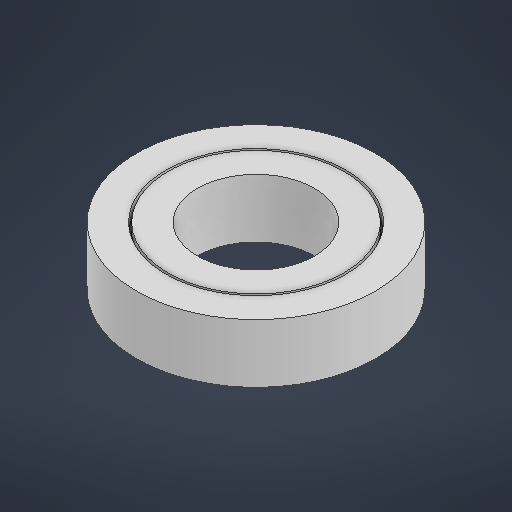
# Autodesk Inventor part: BearingTest
Saved by Autodesk Inventor 2026.1 (Build 301233020, 233B)
## iProperties
Created: 2025-10-08
Part Number: BearingTest
Material: Generic
Document SubType Name: Modeling
Designer: skybound
Density: 1 g/cm^3
Appearance: Default
Author: skybound
Autodesk Inventor part; units mm, degrees
ref_plane "YZ Plane" through (0, 0, 0) normal (1, 0, 0) x (0, 1, 0)
ref_plane "XZ Plane" through (0, 0, 0) normal (0, 1, 0) x (-1, 0, 0)
ref_plane "XY Plane" through (0, 0, 0) normal (0, 0, 1) x (1, 0, 0)
sketch "Sketch1" plane through (0, 0, 0) normal (0, 0, 1) x (1, 0, 0)
  line L0 (0, 0) -> (0, 31.7838) construction
  line L1 (8, 0) -> (8, 8)
  line L2 (8, 8) -> (12, 8)
  line L3 (12, 8) -> (12, 6.6243)
  line L4 (12, 6.6243) -> (10, 4.6243)
  line L5 (10, 4.6243) -> (10, 3.3757)
  line L6 (10, 3.3757) -> (12, 1.3757)
  line L7 (12, 1.3757) -> (12, 0)
  line L8 (12, 0) -> (8, 0)
  line L9 (12.3, 8) -> (12.3, 6.5)
  line L10 (12.3, 6.5) -> (10.3, 4.5)
  line L11 (10.3, 4.5) -> (10.3, 3.5)
  line L12 (10.3, 3.5) -> (12.3, 1.5)
  line L13 (12.3, 1.5) -> (12.3, 0)
  line L14 (16.3, 0) -> (16.3, 8)
  line L15 (16.3, 8) -> (12.3, 8)
  line L16 (12.3, 0) -> (16.3, 0)
  point P0 (11.3, 5.5)
  dimension "d0" = 8
  dimension "d1" = 4
  dimension "d2" = 135
  dimension "d3" = 4
  dimension "d4" = 0.3
  dimension "d5" = 0.3
  dimension "d6" = 0.3
  dimension "d7" = 8
  dimension "d8" = 1.5
  dimension "d9" = 1
  constraints: 34 end point, 9 point on line, 6 parallel, 4 perpendicular, 3 equal length, 3 vertical, 1 midpoint
  measures "d0" distance of L1.start L1.end
  measures "d1" distance of L1.end L2.end
  measures "d2" angle of L3 L4
  measures "d3" distance of L14.end L9.start
  measures "d4" distance between parallel lines of L3 L9
  measures "d5" distance from line of point (11.3, 5.5) L4
  measures "d6" distance between parallel lines of L11 L5
  measures "d7" distance between parallel lines of L0 L1
  measures "d8" distance of L9.start L9.end
  measures "d9" distance of L10.end L11.end
revolve "Revolution1" add sketch "Sketch1" angle 360 about axis through (0, 0, 0) along (0, 1, 0)
equation "\"d5\" = d4"
equation "\"d6\" = d4"
body "Solid1"
